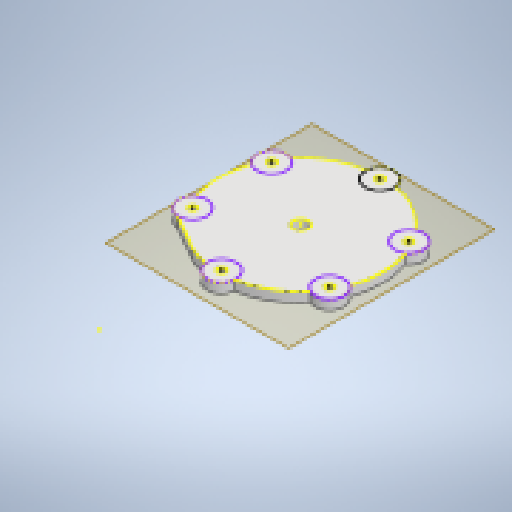
# Autodesk Inventor part: top_cover
Saved by Autodesk Inventor 2023.1 (Build 271208000, 208)
## iProperties
Created: 2024-02-14
Part Number: top_cover
Material: Generic
Document SubType Name: Modeling
Designer: Robot
Density: 1 g/cm^3
Appearance: Default
Author: Robot
Autodesk Inventor part; units mm, degrees
ref_plane "YZ Plane" through (0, 0, 0) normal (1, 0, 0) x (0, 1, 0)
ref_plane "XZ Plane" through (0, 0, 0) normal (0, 1, 0) x (-1, 0, 0)
ref_plane "XY Plane" through (0, 0, 0) normal (0, 0, 1) x (1, 0, 0)
ref_plane "Work Plane1" through (2.7683, 18.8072, -56.8449) normal (0, 1, 0) x (-1, 0, 0)
sketch "Sketch3" plane through (2.7683, 18.8072, -56.8449) normal (0, 1, 0) x (-1, 0, 0)
  circle A0 centre (0, 0) radius 19
  circle A1 centre (0, 0) radius 24.2416
  circle A2 centre (0, 23.4784) radius 1.1
  circle A3 centre (0, 23.4784) radius 4.2925
  circle A4 centre (0, 0) radius 2.25
  circle A5 centre (0, 0) radius 6.5
  line L0 (0, 23.4784) -> (0, 0)
  point P0 (2.7683, 56.8449)
  dimension "d3" = 38
  dimension "d4" = 2.2
  dimension "d5" = 4.5
  dimension "d18" = 13
  constraints: 6 centre point, 4 coincident, 2 end point, 1 vertical
  measures "d3" diameter of A0
  measures "d4" diameter of A2
  measures "d5" diameter of A4
  measures "d18" diameter of A5
extrude "Extrusion2" add sketch "Sketch3" along normal blind 3 contours A0 | A1 A3 | A3 L0 A2 A1 | A1 A2 L0 A3 | A2 A1 | A5 picked at (0, 23.6195)
extrude "Extrusion3" add sketch "Sketch3" along normal blind 5 contours A3 L0 A2 A1 | A1 A2 A3 | A1 A2 L0 A3
pattern_circular "Circular Pattern1" count 6 over 360 about axis through (2.7683, 18.8072, -56.8449) along (0, 1, 0) of "Extrusion3"
extrude "Extrusion4" cut sketch "Sketch3" along normal blind 5 contours A2 A1 | A1 A2
pattern_circular "Circular Pattern2" count 6 over 360 about axis through (2.7683, 18.8072, -56.8449) along (0, 1, 0) of "Extrusion4"
extrude "Extrusion5" add sketch "Sketch3" along normal blind 13 contours A5
sketch "Sketch4" plane through (2.7683, 21.8072, -56.8449) normal (0, 1, 0) x (1, 0, 0)
  circle A0 centre (0, 0) radius 24.2368
  circle A1 centre (0, 0) radius 22.7368
  circle A2 centre (-20.3329, -11.7392) radius 4.2925 projected
  circle A3 centre (-20.3329, 11.7392) radius 4.2925 projected
  circle A4 centre (0, 23.4784) radius 4.2925 projected
  circle A5 centre (20.3329, 11.7392) radius 4.2925 projected
  circle A6 centre (20.3329, -11.7392) radius 4.2925 projected
  circle A7 centre (0, -23.4784) radius 4.2925 projected
  point P0 (-2.7683, -56.8449)
  point P1 (4.1432, -22.3561)
  point P2 (4.2758, -23.8566)
  point P3 (18.5225, -15.6313)
  point P4 (17.2894, -14.7662)
  point P5 (21.4325, -7.5899)
  point P6 (22.7984, -8.2254)
  point P7 (22.7984, 8.2254)
  point P8 (21.4325, 7.5899)
  point P9 (17.2894, 14.7662)
  point P10 (18.5225, 15.6313)
  point P11 (4.2758, 23.8566)
  point P12 (4.1432, 22.3561)
  point P13 (-4.1432, 22.3561)
  point P14 (-4.2758, 23.8566)
  point P15 (-18.5225, 15.6313)
  point P16 (-17.2894, 14.7662)
  point P17 (-21.4325, 7.5899)
  point P18 (-22.7984, 8.2254)
  point P19 (-22.7984, -8.2254)
  point P20 (-21.4325, -7.5899)
  point P21 (-4.2758, -23.8566)
  point P22 (-4.1432, -22.3561)
  point P23 (-17.2894, -14.7662)
  point P24 (-18.5225, -15.6313)
  dimension "d21" = 1.5
  constraints: 2 centre point, 1 coincident
  measures "d21" radial gap between concentric circles of A0 A1
extrude "Extrusion6" add sketch "Sketch4" along normal up to surface (2 mm away) contours A0 A6 A1 A5 | A5 A1 A4 A0 | A0 A7 A1 A6 | A4 A1 A3 A0 | A0 A2 A1 A7 | A3 A1 A2 A0
ref_plane "Work Plane2" through (2.7683, 23.8072, -33.3665) normal (1, 0, 0) x (0, -1, 0)
sketch "Sketch5" plane through (2.7683, 23.8072, -33.3665) normal (1, 0, 0) x (0, -1, 0)
  line L0 (2, 4.2925) -> (0, 4.2925) projected
  line L1 (2, 16.9784) -> (-8, 16.9784) projected
  line L2 (0.7966, 2.2925) -> (1.9512, 2.2925)
  line L3 (1.9512, 18.9784) -> (-6.7913, 18.9784)
  line L4 (0.7966, 2.2925) -> (-6.7913, 18.9784)
  line L5 (1.9512, 18.9784) -> (1.9512, 2.2925)
  point P0 (23.8072, -33.3665)
  point P1 (-6.3354, 16.9784)
  point P2 (1, 4.2925)
  point P3 (-3, 16.9784)
  point P4 (1.9512, 16.9784)
  point P5 (-5.8818, 16.9784)
  dimension "d26" = 2
  dimension "d27" = 2
  constraints: 8 end point, 2 horizontal, 2 midpoint, 1 point on line, 1 vertical
  measures "d26" distance from line of L2 point (1, 4.293)
  measures "d27" distance from line of point (-3, 16.978) L3
extrude "Extrusion8" add sketch "Sketch5" along normal mid plane 2
pattern_circular "Circular Pattern3" count 6 over 360 about axis through (2.7683, 18.8072, -56.8449) along (0, 1, 0) of "Extrusion8"
sketch "Sketch6" plane through (2.7683, 23.8072, -56.8449) normal (0, 1, 0) x (1, 0, 0)
  circle A0 centre (0, -23.4784) radius 1.1 projected
  circle A1 centre (0, -23.4784) radius 4.2925
  point P0 (-2.7683, -56.8449)
  constraints: 1 centre point, 1 coincident
extrude "Extrusion9" cut sketch "Sketch6" along normal blind 4.75
pattern_circular "Circular Pattern4" count 6 over 360 about axis through (2.7683, 18.8072, -56.8449) along (0, 1, 0) of "Extrusion9"
chamfer "Chamfer1" distance 1.5 angle 45 6 edges at (-18.1146, 23.8072, -67.6315) (1.6683, 23.8072, -80.3233) (22.5512, 23.8072, -69.5368) (23.6512, 23.8072, -46.0584) (3.8683, 23.8072, -33.3665) (-17.0146, 23.8072, -44.1531)
chamfer "Chamfer2" distance 4 angle 45 1 edges at (9.2683, 21.8072, -56.8449)
chamfer "Chamfer3" distance 4 angle 45 1 edges at (5.0183, 18.8072, -56.8449)
body "Solid2"
